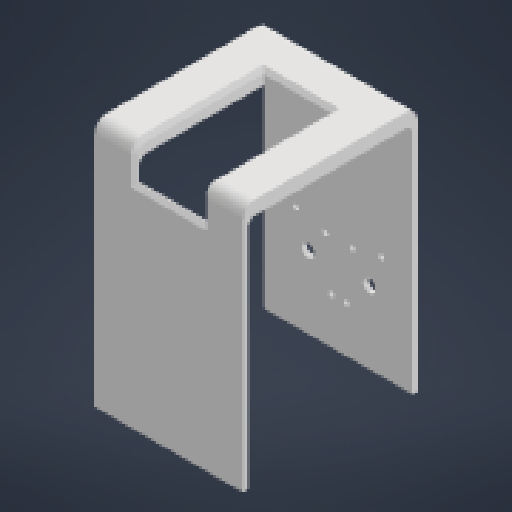
# Autodesk Inventor part: Head_Box_Base
Saved by Autodesk Inventor 2024 (Build 280153000, 153)
## iProperties
Created: 2025-09-22
Part Number: Head_Box_Base
Material: Generic
Document SubType Name: Modeling
Designer: kevin
Density: 1 g/cm^3
Appearance: Default
Author: kevin
Autodesk Inventor part; units mm, degrees
ref_plane "YZ Plane" through (0, 0, 0) normal (1, 0, 0) x (0, 1, 0)
ref_plane "XZ Plane" through (0, 0, 0) normal (0, 1, 0) x (-1, 0, 0)
ref_plane "XY Plane" through (0, 0, 0) normal (0, 0, 1) x (1, 0, 0)
sketch "Sketch1" plane through (0, 0, 0) normal (0, 0, 1) x (1, 0, 0)
  circle A0 centre (57.1655, 18.417) radius 2.1 projected
  circle A1 centre (12.7885, 12.5269) radius 2.1 projected
  circle A2 centre (17.2869, -26.8107) radius 2.1 projected
  circle A3 centre (-1.1004, -6.0436) radius 5 projected
  line L0 (64.4194, 6.1067) -> (62.3371, -1.6056) projected
  line L1 (67.3095, 9.3686) -> (64.4194, 6.1067) projected
  ellipse E0 centre (57.1655, 18.417) end of major axis (47.0979, 27.5508) minor radius 11.51 (67.3095, 9.3686) -> (68.6853, 21.7358) ccw projected
  ellipse E1 centre (54.4602, 15.4351) end of major axis (43.6731, 3.5452) minor radius 13.5934 (68.6853, 21.7358) -> (59.3507, 30.2045) ccw projected
  ellipse E2 centre (57.1655, 18.417) end of major axis (47.0979, 27.5508) minor radius 11.51 (59.3507, 30.2045) -> (47.0214, 27.4655) ccw projected
  line L2 (36.5043, 15.5956) -> (47.0214, 27.4655) projected
  arc A4 (36.5043, 15.5956) -> (29.6862, 12.4398) centre (33.7853, 12.5269) ccw projected
  line L3 (16.8875, 12.4398) -> (29.6862, 12.4398) projected
  arc A5 (16.8875, 12.4398) -> (10.0695, 15.5956) centre (12.7885, 12.5269) ccw projected
  line L4 (10.0695, 15.5956) -> (-0.4476, 27.4655) projected
  ellipse E3 centre (-10.5917, 18.417) end of major axis (-0.5241, 27.5508) minor radius 11.51 (-0.4476, 27.4655) -> (-12.7769, 30.2045) ccw projected
  ellipse E4 centre (-7.8864, 15.4351) end of major axis (2.9006, 3.5452) minor radius 13.5934 (-12.7769, 30.2045) -> (-22.1115, 21.7358) ccw projected
  ellipse E5 centre (-10.5917, 18.417) end of major axis (-0.5241, 27.5508) minor radius 11.51 (-22.1115, 21.7358) -> (-20.7358, 9.3686) ccw projected
  line L5 (-20.7358, 9.3686) -> (-17.8456, 6.1067) projected
  line L6 (-17.8456, 6.1067) -> (-15.7633, -1.6056) projected
  line L7 (-15.7633, -1.6056) -> (-6.4546, -11.2249) projected
  line L8 (-6.4546, -11.2249) -> (1.9738, -21.6241) projected
  line L9 (1.9738, -21.6241) -> (9.6038, -24.7107) projected
  line L10 (9.6038, -24.7107) -> (14.4693, -29.7892) projected
  arc A6 (14.4693, -29.7892) -> (17.2869, -30.9107) centre (17.2869, -26.8107) ccw projected
  line L11 (17.2869, -30.9107) -> (29.2869, -30.9107) projected
  arc A7 (29.2869, -30.9107) -> (32.1045, -29.7892) centre (29.2869, -26.8107) ccw projected
  line L12 (36.97, -24.7107) -> (32.1045, -29.7892) projected
  line L13 (44.6, -21.6241) -> (36.97, -24.7107) projected
  line L14 (53.0284, -11.2249) -> (44.6, -21.6241) projected
  line L15 (62.3371, -1.6056) -> (53.0284, -11.2249) projected
  circle A8 centre (-10.5917, 18.417) radius 2.1 projected
  circle A9 centre (47.6742, -6.0436) radius 5 projected
  circle A10 centre (29.2869, -26.8107) radius 2.1 projected
  circle A11 centre (33.7853, 12.5269) radius 2.1 projected
  arc A12 (-51.3703, 45.0767) -> (97.4441, 45.0767) centre (23.0369, 31.7099) ccw construction
  arc A13 (51.5869, 99.9923) -> (-5.5131, 99.9923) centre (23.0369, 31.7099) ccw construction
  arc A14 (-50.582, -28.3339) -> (101.2571, -22.203) centre (23.0369, 31.7099) ccw construction
  line L16 (23.0369, 31.7099) -> (23.2869, -30.9107) construction
  line L17 (85.5258, 132.2899) -> (-39.4742, 132.2899)
  line L18 (-39.4742, 132.2899) -> (-39.4742, -63.2901)
  line L19 (-39.4742, -63.2901) -> (85.5258, -63.2901)
  line L20 (85.5258, -63.2901) -> (85.5258, 132.2899)
  line L21 (85.5258, 132.2899) -> (-39.4742, -63.2901) construction
  line L22 (-39.4742, 132.2899) -> (85.5258, -63.2901) construction
  point P0 (0, 0)
  point P1 (23.0258, 34.4999)
  dimension "d0" = 195.58
  dimension "d27" = 125
  constraints: 14 end point, 3 midpoint, 2 parallel, 1 horizontal, 1 perpendicular, 1 point on line, 1 tangent, 6 other
  measures "d0" distance of L17.end L18.end
  measures "d27" distance of L17.start L17.end
extrude "Extrusion1" add sketch "Sketch1" along normal blind 4 contours L0 L15 L14 L13 L12 A7 L11 A6 L10 L9 L8 L7 L6 L5 E5 E4 E3 L4 A5 L3 A4 L2 E2 E1 E0 L1 | L20 L19 L18 L17
sketch "Sketch2" plane through (0, 0, 4) normal (0, 0, 1) x (1, 0, 0)
  line L0 (-39.4742, 132.2899) -> (-39.4742, -63.2901) projected
  line L1 (-39.4742, -63.2901) -> (85.5258, -63.2901) projected
  line L2 (85.5258, -63.2901) -> (85.5258, 132.2899) projected
  line L3 (85.5258, 132.2899) -> (-39.4742, 132.2899) projected
  circle A0 centre (12.7885, 12.5269) radius 2.1 projected
  circle A1 centre (33.7853, 12.5269) radius 2.1 projected
  circle A2 centre (29.2869, -26.8107) radius 2.1 projected
  circle A3 centre (47.6742, -6.0436) radius 5 projected
  circle A4 centre (-10.5917, 18.417) radius 2.1 projected
  circle A5 centre (-1.1004, -6.0436) radius 5 projected
  circle A6 centre (17.2869, -26.8107) radius 2.1 projected
  circle A7 centre (57.1655, 18.417) radius 2.1 projected
  line L4 (85.5258, 132.2899) -> (-39.4742, 132.2899)
  line L5 (-39.4742, 132.2899) -> (-39.4742, 127.2899)
  line L6 (-39.4742, 127.2899) -> (85.5258, 127.2899)
  line L7 (85.5258, 127.2899) -> (85.5258, 132.2899)
  line L8 (52.5258, 127.2899) -> (-6.4742, 127.2899)
  line L9 (-6.4742, 127.2899) -> (-6.4742, 133.2899)
  line L10 (-6.4742, 133.2899) -> (52.5258, 133.2899)
  line L11 (52.5258, 133.2899) -> (52.5258, 127.2899)
  point P0 (0, 0)
  point P1 (-39.4742, 127.2899)
  point P2 (85.5258, 127.2899)
  dimension "d3" = 5
  dimension "d7" = 6
  dimension "d8" = 33
  dimension "d9" = 33
  constraints: 16 end point, 4 parallel, 2 horizontal, 2 perpendicular, 1 collinear, 1 point on line
  measures "d3" distance of L5.end L4.end
  measures "d7" distance of L10.end L8.start
  measures "d8" distance between parallel lines of L2 L11
  measures "d9" distance between parallel lines of L0 L9
extrude "Extrusion2" add sketch "Sketch2" along normal blind 130 contours L3 L9 L6 L0 | L3 L11 L6 L9 | L3 L2 L6 L11
sketch "Sketch4" plane through (0, 0, 134) normal (0, 0, 1) x (1, 0, 0)
  line L0 (85.5258, 127.2899) -> (-39.4742, 127.2899) projected
  line L1 (-39.4742, 127.2899) -> (-39.4742, -63.2901) projected
  line L2 (-39.4742, -63.2901) -> (85.5258, -63.2901) projected
  line L3 (85.5258, -63.2901) -> (85.5258, 127.2899) projected
  circle A0 centre (12.7885, 12.5269) radius 2.1 projected
  circle A1 centre (33.7853, 12.5269) radius 2.1 projected
  circle A2 centre (29.2869, -26.8107) radius 2.1 projected
  circle A3 centre (47.6742, -6.0436) radius 5 projected
  circle A4 centre (-10.5917, 18.417) radius 2.1 projected
  circle A5 centre (-1.1004, -6.0436) radius 5 projected
  circle A6 centre (17.2869, -26.8107) radius 2.1 projected
  circle A7 centre (57.1655, 18.417) radius 2.1 projected
  line L4 (85.5258, 127.2899) -> (85.5258, 132.2899) projected
  line L5 (85.5258, 132.2899) -> (-39.4742, 132.2899) projected
  line L6 (-39.4742, 132.2899) -> (-39.4742, 127.2899) projected
  line L7 (-39.4742, 127.2899) -> (85.5258, 127.2899) projected
  point P0 (0, 0)
extrude "Extrusion3" add sketch "Sketch4" along normal blind 4 contours L3 L2 L1 L0 | L0 L6 L5 L4 | A0 | A1 | A2 | A3 | A4 | A5 | A6 | A7
fillet "Fillet1" [suppressed]
sketch "Sketch6" plane through (0, 0, 138) normal (0, 0, 1) x (1, 0, 0)
  line L0 (85.5258, 132.2899) -> (-39.4742, 132.2899) projected
  line L1 (-39.4742, 132.2899) -> (-39.4742, -63.2901) projected
  line L2 (-39.4742, -63.2901) -> (85.5258, -63.2901) projected
  line L3 (85.5258, -63.2901) -> (85.5258, 132.2899) projected
  line L4 (48.5258, 138.9893) -> (-2.4742, 138.9893)
  line L5 (-2.4742, 138.9893) -> (-2.4742, 104.2541)
  line L6 (-2.4742, 104.2541) -> (48.5258, 104.2541)
  line L7 (48.5258, 104.2541) -> (48.5258, 138.9893)
  point P0 (0, 0)
  dimension "d16" = 37
  dimension "d17" = 37
  constraints: 8 end point, 2 parallel, 1 horizontal, 1 perpendicular
  measures "d16" distance between parallel lines of L3 L7
  measures "d17" distance between parallel lines of L5 L1
extrude "Extrusion5" cut sketch "Sketch6" against normal blind 101.6 contours L7 L6 L5 L0 | L0 L5 L4 L7
fillet "Fillet2" radius 9.525 5 edges at (67.0258, 132.2899, 138) (-20.9742, 132.2899, 138) (23.0258, 132.2899, 0) (-20.9742, 127.2899, 134) (67.0258, 127.2899, 134)
chamfer "Chamfer1" distance 3.175 angle 45 8 edges at (23.0258, 132.2899, 36.4) (48.5258, 132.2899, 82.4375) (48.5258, 129.5001, 135.2102) (48.5258, 113.5095, 138) (-2.4742, 132.2899, 82.4375) (-2.4742, 129.5001, 135.2102) (-2.4742, 113.5095, 138) (23.0258, 104.2541, 138)
chamfer "Chamfer2" distance 4 angle 45 1 edges at (23.0258, 127.2899, 4)
equation "\"d9\" = d8"
equation "\"d17\" = d16"
body "Solid1"
